Cyclone  Cyclone to Vacuum Adapter (Autodesk Fusion 360 design; units mm, degrees)
Autodesk Fusion 360 part; units mm, degrees
sketch "Sketch2" plane through (0, 0, 0) normal (0, 1, 0) x (1, 0, 0)
  circle A0 centre (0, 0) radius 24
  circle A1 centre (0, 0) radius 25.25
  circle A2 centre (0, 0) radius 27
  dimension "d6" = 48
  dimension "d29" = 50.5
  dimension "d37" = 54
  constraint coincident A0.centre A1.centre
  measures "d6" diameter of A0
  measures "d29" diameter of A1
  measures "d37" diameter of A2
extrude "Extrude1" add sketch "Sketch2" along normal blind 31 contours A2
sketch "Sketch3" plane through (0, 0, 0) normal (1, 0, 0) x (0, 0, -1)
  ellipse E0 centre (0, 14.5) end of major axis (-6.75, 14.5) minor radius 4.5
  line L0 (6.75, 14.5) -> (-6.75, 14.5)
  line L1 (0, 19) -> (0, 10)
  dimension "d18" = 13.5
  dimension "d20" = 14.5
  dimension "d49" = 4.5
  constraint horizontal L0
  constraint coincident E0 L0.start
  constraint coincident E0 L0.end
  constraint coincident E0 L1.start
  constraint coincident E0 L1.end
  measures "d18" distance of E0
  measures "d20" distance of origin E0.centre
  measures "d49" distance of E0.centre L1.end
extrude "Extrude8" cut sketch "Sketch3" along normal mid plane 60
ref_plane "WorkPlane3" through (0, 27.5, 0) normal (0, -1, 0) x (-1, 0, 0)
ref_plane "WorkPlane4" through (0, 52.5, 0) normal (0, -1, 0) x (-1, 0, 0)
sketch "Sketch7" plane through (0, 52.5, 0) normal (0, -1, 0) x (1, 0, 0)
  circle A0 centre (0, 0) radius 23
  circle A1 centre (0, 0) radius 24.5
  dimension "d63" = 46
  dimension "d64" = 49
  constraint coincident A0.centre A1.centre
  measures "d63" diameter of A0
  measures "d64" diameter of A1
sketch "Sketch8" plane through (0, 27.5, 0) normal (0, -1, 0) x (1, 0, 0)
  circle A0 centre (0, 0) radius 25
  circle A1 centre (0, 0) radius 23.5
  circle A2 centre (0, 0) radius 27
  dimension "d67" = 50
  dimension "d68" = 47
  dimension "d76" = 54
  constraint coincident A0.centre A1.centre
  constraint concentric A0 A1
  measures "d67" diameter of A0
  measures "d68" diameter of A1
  measures "d76" diameter of A2
ref_plane "WorkPlane5" through (0, 42.5, 0) normal (0, -1, 0) x (1, 0, 0)
sketch "Sketch10" plane through (0, 42.5, 0) normal (0, -1, 0) x (1, 0, 0)
  circle A0 centre (0, 0) radius 23.5
  circle A1 centre (0, 0) radius 25
  dimension "d70" = 47
  dimension "d71" = 50
  constraint coincident A0.centre A1.centre
  constraint concentric A0 A1
  measures "d70" diameter of A0
  measures "d71" diameter of A1
extrude "Extrude14" add sketch "Sketch8" against normal blind 3.5 contours A0 | A2
extrude "Extrude13" add sketch "Sketch8" against normal blind 15 contours A0
loft "Loft1" add profiles "Sketch10", "Sketch7" section 1 section 2
loft "Loft2" cut profiles "Sketch7", "Sketch10" section 1 contours A0 section 2 contours A0
chamfer "Chamfer5" distance 2 angle 45 1 edges at (-23.3082, 31, -9.0404)
chamfer "Chamfer6" distance 1.75 angle 45 1 edges at (-23.5413, 27.5, 9.1308)
